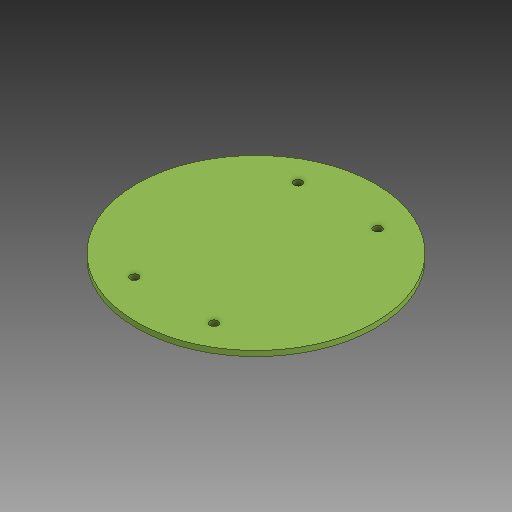
# Autodesk Inventor part: tsop_board
Saved by Autodesk Inventor 2020 (Build 240168000, 168)
## iProperties
Created: 2024-11-04
Part Number: tsop_board
Material: Медь
Document SubType Name: Modeling
Designer: Ivan
Density: 8.94 g/cm^3
Appearance: Оливково-зеленый
Mass: 133.751 g
Surface Area: 157.837 cm^2
Volume: 14.961 cm^3
Author: Ivan
Autodesk Inventor part; units mm, degrees
(part 1 of 2)
ref_plane "YZ Plane" through (0, 0, 0) normal (1, 0, 0) x (0, 1, 0)
ref_plane "XZ Plane" through (0, 0, 0) normal (0, 1, 0) x (-1, 0, 0)
ref_plane "XY Plane" through (0, 0, 0) normal (0, 0, 1) x (1, 0, 0)
sketch "Эскиз1" plane through (0, 0, 0) normal (0, 1, 0) x (-1, 0, 0)
  line L0 (44.0469, 3.6) -> (38.8469, 3.6)
  line L1 (38.8469, 3.6) -> (38.8469, -3.6)
  line L2 (38.8469, -3.6) -> (44.0469, -3.6)
  line L3 (44.0469, -3.6) -> (44.0469, 3.6)
  line L4 (0, 0) -> (38.8469, 0) construction
  circle A0 centre (0, 0) radius 41.603 construction
  line L5 (41.4469, 3.6) -> (41.4469, -3.6) construction
  line L6 (37.3982, 11.1095) -> (38.8028, 4.0478)
  line L7 (42.4983, 12.124) -> (37.3982, 11.1095)
  line L8 (43.9029, 5.0623) -> (42.4983, 12.124)
  line L9 (38.8028, 4.0478) -> (43.9029, 5.0623)
  line L10 (34.5122, 18.192) -> (37.2675, 11.5401)
  line L11 (39.3164, 20.182) -> (34.5122, 18.192)
  line L12 (42.0717, 13.5301) -> (39.3164, 20.182)
  line L13 (37.2675, 11.5401) -> (42.0717, 13.5301)
  line L14 (30.3, 24.5755) -> (34.3001, 18.5889)
  line L15 (34.6236, 27.4645) -> (30.3, 24.5755)
  line L16 (38.6237, 21.4779) -> (34.6236, 27.4645)
  line L17 (34.3001, 18.5889) -> (38.6237, 21.4779)
  line L18 (24.9233, 30.0145) -> (30.0145, 24.9233)
  line L19 (28.6003, 33.6915) -> (24.9233, 30.0145)
  line L20 (33.6915, 28.6003) -> (28.6003, 33.6915)
  line L21 (30.0145, 24.9233) -> (33.6915, 28.6003)
  line L22 (18.5889, 34.3001) -> (24.5755, 30.3)
  line L23 (21.4779, 38.6237) -> (18.5889, 34.3001)
  line L24 (27.4645, 34.6236) -> (21.4779, 38.6237)
  line L25 (24.5755, 30.3) -> (27.4645, 34.6236)
  line L26 (11.5401, 37.2675) -> (18.192, 34.5122)
  line L27 (13.5301, 42.0717) -> (11.5401, 37.2675)
  line L28 (20.182, 39.3164) -> (13.5301, 42.0717)
  line L29 (18.192, 34.5122) -> (20.182, 39.3164)
  line L30 (4.0478, 38.8028) -> (11.1095, 37.3982)
  line L31 (5.0623, 43.9029) -> (4.0478, 38.8028)
  line L32 (12.124, 42.4983) -> (5.0623, 43.9029)
  line L33 (11.1095, 37.3982) -> (12.124, 42.4983)
  line L34 (-3.6, 38.8469) -> (3.6, 38.8469)
  line L35 (-3.6, 44.0469) -> (-3.6, 38.8469)
  line L36 (3.6, 44.0469) -> (-3.6, 44.0469)
  line L37 (3.6, 38.8469) -> (3.6, 44.0469)
  line L38 (-11.1095, 37.3982) -> (-4.0478, 38.8028)
  line L39 (-12.124, 42.4983) -> (-11.1095, 37.3982)
  line L40 (-5.0623, 43.9029) -> (-12.124, 42.4983)
  line L41 (-4.0478, 38.8028) -> (-5.0623, 43.9029)
  line L42 (-18.192, 34.5122) -> (-11.5401, 37.2675)
  line L43 (-20.182, 39.3164) -> (-18.192, 34.5122)
  line L44 (-13.5301, 42.0717) -> (-20.182, 39.3164)
  line L45 (-11.5401, 37.2675) -> (-13.5301, 42.0717)
  line L46 (-24.5755, 30.3) -> (-18.5889, 34.3001)
  line L47 (-27.4645, 34.6236) -> (-24.5755, 30.3)
  line L48 (-21.4779, 38.6237) -> (-27.4645, 34.6236)
  line L49 (-18.5889, 34.3001) -> (-21.4779, 38.6237)
  line L50 (-30.0145, 24.9233) -> (-24.9233, 30.0145)
  line L51 (-33.6915, 28.6003) -> (-30.0145, 24.9233)
  line L52 (-28.6003, 33.6915) -> (-33.6915, 28.6003)
  line L53 (-24.9233, 30.0145) -> (-28.6003, 33.6915)
  line L54 (-34.3001, 18.5889) -> (-30.3, 24.5755)
  line L55 (-38.6237, 21.4779) -> (-34.3001, 18.5889)
  line L56 (-34.6236, 27.4645) -> (-38.6237, 21.4779)
  line L57 (-30.3, 24.5755) -> (-34.6236, 27.4645)
  line L58 (-37.2675, 11.5401) -> (-34.5122, 18.192)
  line L59 (-42.0717, 13.5301) -> (-37.2675, 11.5401)
  line L60 (-39.3164, 20.182) -> (-42.0717, 13.5301)
  line L61 (-34.5122, 18.192) -> (-39.3164, 20.182)
  line L62 (-38.8028, 4.0478) -> (-37.3982, 11.1095)
  line L63 (-43.9029, 5.0623) -> (-38.8028, 4.0478)
  line L64 (-42.4983, 12.124) -> (-43.9029, 5.0623)
  line L65 (-37.3982, 11.1095) -> (-42.4983, 12.124)
  line L66 (-38.8469, -3.6) -> (-38.8469, 3.6)
  line L67 (-44.0469, -3.6) -> (-38.8469, -3.6)
  line L68 (-44.0469, 3.6) -> (-44.0469, -3.6)
  line L69 (-38.8469, 3.6) -> (-44.0469, 3.6)
  line L70 (-37.3982, -11.1095) -> (-38.8028, -4.0478)
  line L71 (-42.4983, -12.124) -> (-37.3982, -11.1095)
  line L72 (-43.9029, -5.0623) -> (-42.4983, -12.124)
  line L73 (-38.8028, -4.0478) -> (-43.9029, -5.0623)
  line L74 (-34.5122, -18.192) -> (-37.2675, -11.5401)
  line L75 (-39.3164, -20.182) -> (-34.5122, -18.192)
  line L76 (-42.0717, -13.5301) -> (-39.3164, -20.182)
  line L77 (-37.2675, -11.5401) -> (-42.0717, -13.5301)
  line L78 (-30.3, -24.5755) -> (-34.3001, -18.5889)
  line L79 (-34.6236, -27.4645) -> (-30.3, -24.5755)
  line L80 (-38.6237, -21.4779) -> (-34.6236, -27.4645)
  line L81 (-34.3001, -18.5889) -> (-38.6237, -21.4779)
  line L82 (-24.9233, -30.0145) -> (-30.0145, -24.9233)
  line L83 (-28.6003, -33.6915) -> (-24.9233, -30.0145)
  line L84 (-33.6915, -28.6003) -> (-28.6003, -33.6915)
  line L85 (-30.0145, -24.9233) -> (-33.6915, -28.6003)
  line L86 (-18.5889, -34.3001) -> (-24.5755, -30.3)
  line L87 (-21.4779, -38.6237) -> (-18.5889, -34.3001)
  line L88 (-27.4645, -34.6236) -> (-21.4779, -38.6237)
  line L89 (-24.5755, -30.3) -> (-27.4645, -34.6236)
  line L90 (-11.5401, -37.2675) -> (-18.192, -34.5122)
  line L91 (-13.5301, -42.0717) -> (-11.5401, -37.2675)
  line L92 (-20.182, -39.3164) -> (-13.5301, -42.0717)
  line L93 (-18.192, -34.5122) -> (-20.182, -39.3164)
  line L94 (-4.0478, -38.8028) -> (-11.1095, -37.3982)
  line L95 (-5.0623, -43.9029) -> (-4.0478, -38.8028)
  line L96 (-12.124, -42.4983) -> (-5.0623, -43.9029)
  line L97 (-11.1095, -37.3982) -> (-12.124, -42.4983)
  line L98 (3.6, -38.8469) -> (-3.6, -38.8469)
  line L99 (3.6, -44.0469) -> (3.6, -38.8469)
  line L100 (-3.6, -44.0469) -> (3.6, -44.0469)
  line L101 (-3.6, -38.8469) -> (-3.6, -44.0469)
  line L102 (11.1095, -37.3982) -> (4.0478, -38.8028)
  line L103 (12.124, -42.4983) -> (11.1095, -37.3982)
  line L104 (5.0623, -43.9029) -> (12.124, -42.4983)
  line L105 (4.0478, -38.8028) -> (5.0623, -43.9029)
  line L106 (18.192, -34.5122) -> (11.5401, -37.2675)
  line L107 (20.182, -39.3164) -> (18.192, -34.5122)
  line L108 (13.5301, -42.0717) -> (20.182, -39.3164)
  line L109 (11.5401, -37.2675) -> (13.5301, -42.0717)
  line L110 (24.5755, -30.3) -> (18.5889, -34.3001)
  line L111 (27.4645, -34.6236) -> (24.5755, -30.3)
  line L112 (21.4779, -38.6237) -> (27.4645, -34.6236)
  line L113 (18.5889, -34.3001) -> (21.4779, -38.6237)
  line L114 (30.0145, -24.9233) -> (24.9233, -30.0145)
  line L115 (33.6915, -28.6003) -> (30.0145, -24.9233)
  line L116 (28.6003, -33.6915) -> (33.6915, -28.6003)
  line L117 (24.9233, -30.0145) -> (28.6003, -33.6915)
  line L118 (34.3001, -18.5889) -> (30.3, -24.5755)
  line L119 (38.6237, -21.4779) -> (34.3001, -18.5889)
  line L120 (34.6236, -27.4645) -> (38.6237, -21.4779)
  line L121 (30.3, -24.5755) -> (34.6236, -27.4645)
  line L122 (37.2675, -11.5401) -> (34.5122, -18.192)
  line L123 (42.0717, -13.5301) -> (37.2675, -11.5401)
  line L124 (39.3164, -20.182) -> (42.0717, -13.5301)
  line L125 (34.5122, -18.192) -> (39.3164, -20.182)
  line L126 (38.8028, -4.0478) -> (37.3982, -11.1095)
  line L127 (43.9029, -5.0623) -> (38.8028, -4.0478)
  line L128 (42.4983, -12.124) -> (43.9029, -5.0623)
  line L129 (37.3982, -11.1095) -> (42.4983, -12.124)
  line L130 (38.8028, 4.0478) -> (38.8469, 3.6) construction
  line L131 (38.8469, 3.6) -> (43.9777, 4.1053) construction
  line L132 (43.9029, 5.0623) -> (37.3982, 11.1095) construction
  line L133 (42.4983, 12.124) -> (38.8028, 4.0478) construction
  circle A1 centre (0, 0) radius 41.4469 construction
  line L134 (39.3164, 20.182) -> (37.2675, 11.5401) construction
  line L135 (34.5122, 18.192) -> (42.0717, 13.5301) construction
  line L136 (38.292, 15.8611) -> (0, 0) construction
  line L137 (0, 0) -> (40.6505, 8.0859) construction
  point P0 (41.603, 0)
  point P1 (38.1005, 7.5787)
  point P2 (39.9482, 11.6167)
  point P3 (41.3529, 4.5551)
  point P4 (35.8899, 14.8661)
  point P5 (36.9143, 19.187)
  point P6 (39.6696, 12.5351)
  point P7 (32.3, 21.5822)
  point P8 (32.4618, 26.02)
  point P9 (36.4619, 20.0334)
  point P10 (27.4689, 27.4689)
  point P11 (26.7618, 31.853)
  point P12 (31.853, 26.7618)
  point P13 (21.5822, 32.3)
  point P14 (20.0334, 36.4619)
  point P15 (26.02, 32.4618)
  point P16 (14.8661, 35.8899)
  point P17 (12.5351, 39.6696)
  point P18 (19.187, 36.9143)
  point P19 (7.5787, 38.1005)
  point P20 (4.5551, 41.3529)
  point P21 (11.6167, 39.9482)
  point P22 (0, 38.8469)
  point P23 (-3.6, 41.4469)
  point P24 (3.6, 41.4469)
  point P25 (-7.5787, 38.1005)
  point P26 (-11.6167, 39.9482)
  point P27 (-4.5551, 41.3529)
  point P28 (-14.8661, 35.8899)
  point P29 (-19.187, 36.9143)
  point P30 (-12.5351, 39.6696)
  point P31 (-21.5822, 32.3)
  point P32 (-26.02, 32.4618)
  point P33 (-20.0334, 36.4619)
  point P34 (-27.4689, 27.4689)
  point P35 (-31.853, 26.7618)
  point P36 (-26.7618, 31.853)
  point P37 (-32.3, 21.5822)
  point P38 (-36.4619, 20.0334)
  point P39 (-32.4618, 26.02)
  point P40 (-35.8899, 14.8661)
  point P41 (-39.6696, 12.5351)
  point P42 (-36.9143, 19.187)
  point P43 (-38.1005, 7.5787)
  point P44 (-41.3529, 4.5551)
  point P45 (-39.9482, 11.6167)
  point P46 (-38.8469, 0)
  point P47 (-41.4469, -3.6)
  point P48 (-41.4469, 3.6)
  point P49 (-38.1005, -7.5787)
  point P50 (-39.9482, -11.6167)
  point P51 (-41.3529, -4.5551)
  point P52 (-35.8899, -14.8661)
  point P53 (-36.9143, -19.187)
  point P54 (-39.6696, -12.5351)
  point P55 (-32.3, -21.5822)
  point P56 (-32.4618, -26.02)
  point P57 (-36.4619, -20.0334)
  point P58 (-27.4689, -27.4689)
  point P59 (-26.7618, -31.853)
  point P60 (-31.853, -26.7618)
  point P61 (-21.5822, -32.3)
  point P62 (-20.0334, -36.4619)
  point P63 (-26.02, -32.4618)
  point P64 (-14.8661, -35.8899)
  point P65 (-12.5351, -39.6696)
  point P66 (-19.187, -36.9143)
  point P67 (-7.5787, -38.1005)
  point P68 (-4.5551, -41.3529)
  point P69 (-11.6167, -39.9482)
  point P70 (0, -38.8469)
  point P71 (3.6, -41.4469)
  point P72 (-3.6, -41.4469)
  point P73 (7.5787, -38.1005)
  point P74 (11.6167, -39.9482)
  point P75 (4.5551, -41.3529)
  point P76 (14.8661, -35.8899)
  point P77 (19.187, -36.9143)
  point P78 (12.5351, -39.6696)
  point P79 (21.5822, -32.3)
  point P80 (26.02, -32.4618)
  point P81 (20.0334, -36.4619)
  point P82 (27.4689, -27.4689)
  point P83 (31.853, -26.7618)
  point P84 (26.7618, -31.853)
  point P85 (32.3, -21.5822)
  point P86 (36.4619, -20.0334)
  point P87 (32.4618, -26.02)
  point P88 (35.8899, -14.8661)
  point P89 (39.6696, -12.5351)
  point P90 (36.9143, -19.187)
  point P91 (38.1005, -7.5787)
  point P92 (41.3529, -4.5551)
  point P93 (39.9482, -11.6167)
sketch "Эскиз3" plane through (0, 0, 0) normal (0, 1, 0) x (-1, 0, 0)
  line L0 (38.8028, 4.0478) -> (38.8469, 3.6) construction
  line L1 (38.8249, 3.8239) -> (46.4311, 4.5731) construction
  line L2 (44.0469, -3.6) -> (44.0469, 3.6)
  line L3 (44.0469, -0.05) -> (44.0469, 0.05)
  line L4 (44.0469, 2.45) -> (45.2469, 2.45) construction
  arc A0 (44.0469, 0.05) -> (45.2469, 2.45) centre (42.2469, 2.45) ccw
  line L5 (45.2469, 2.45) -> (45.2469, 0) construction
  line L6 (0, 0) -> (38.8469, 0) construction
  arc A1 (45.2469, -2.45) -> (44.0469, -0.05) centre (42.2469, -2.45) ccw
  arc A2 (43.1908, 8.6422) -> (43.8996, 11.2302) centre (40.9572, 10.6449) ccw
  arc A3 (44.8555, 6.4243) -> (43.2103, 8.5441) centre (41.9131, 5.839) ccw
  line L7 (43.2103, 8.5441) -> (43.1908, 8.6422)
  arc A4 (40.6749, 16.9022) -> (40.8651, 19.5788) centre (38.0935, 18.4307) ccw
  arc A5 (42.7403, 15.0517) -> (40.7132, 16.8098) centre (39.9686, 13.9037) ccw
  line L8 (40.7132, 16.8098) -> (40.6749, 16.9022)
  arc A6 (36.5959, 24.5127) -> (36.2603, 27.1749) centre (33.7659, 25.5082) ccw
  arc A7 (38.9826, 23.1007) -> (36.6515, 24.4296) centre (36.4882, 21.434) ccw
  line L9 (36.6515, 24.4296) -> (36.5959, 24.5127)
  arc A8 (31.1105, 31.1812) -> (30.262, 33.7268) centre (28.1407, 31.6055) ccw
  arc A9 (33.7268, 30.262) -> (31.1812, 31.1105) centre (31.6055, 28.1407) ccw
  line L10 (31.1812, 31.1105) -> (31.1105, 31.1812)
  arc A10 (24.4296, 36.6515) -> (23.1007, 38.9826) centre (21.434, 36.4882) ccw
  arc A11 (27.1749, 36.2603) -> (24.5127, 36.5959) centre (25.5082, 33.7659) ccw
  line L11 (24.5127, 36.5959) -> (24.4296, 36.6515)
  arc A12 (16.8098, 40.7132) -> (15.0517, 42.7403) centre (13.9037, 39.9686) ccw
  arc A13 (19.5788, 40.8651) -> (16.9022, 40.6749) centre (18.4307, 38.0935) ccw
  line L12 (16.9022, 40.6749) -> (16.8098, 40.7132)
  arc A14 (8.5441, 43.2103) -> (6.4243, 44.8555) centre (5.839, 41.9131) ccw
  arc A15 (11.2302, 43.8996) -> (8.6422, 43.1908) centre (10.6449, 40.9572) ccw
  line L13 (8.6422, 43.1908) -> (8.5441, 43.2103)
  arc A16 (-0.05, 44.0469) -> (-2.45, 45.2469) centre (-2.45, 42.2469) ccw
  arc A17 (2.45, 45.2469) -> (0.05, 44.0469) centre (2.45, 42.2469) ccw
  line L14 (0.05, 44.0469) -> (-0.05, 44.0469)
  arc A18 (-8.6422, 43.1908) -> (-11.2302, 43.8996) centre (-10.6449, 40.9572) ccw
  arc A19 (-6.4243, 44.8555) -> (-8.5441, 43.2103) centre (-5.839, 41.9131) ccw
  line L15 (-8.5441, 43.2103) -> (-8.6422, 43.1908)
  arc A20 (-16.9022, 40.6749) -> (-19.5788, 40.8651) centre (-18.4307, 38.0935) ccw
  arc A21 (-15.0517, 42.7403) -> (-16.8098, 40.7132) centre (-13.9037, 39.9686) ccw
  line L16 (-16.8098, 40.7132) -> (-16.9022, 40.6749)
  arc A22 (-24.5127, 36.5959) -> (-27.1749, 36.2603) centre (-25.5082, 33.7659) ccw
  arc A23 (-23.1007, 38.9826) -> (-24.4296, 36.6515) centre (-21.434, 36.4882) ccw
  line L17 (-24.4296, 36.6515) -> (-24.5127, 36.5959)
  arc A24 (-31.1812, 31.1105) -> (-33.7268, 30.262) centre (-31.6055, 28.1407) ccw
  arc A25 (-30.262, 33.7268) -> (-31.1105, 31.1812) centre (-28.1407, 31.6055) ccw
  line L18 (-31.1105, 31.1812) -> (-31.1812, 31.1105)
  arc A26 (-36.6515, 24.4296) -> (-38.9826, 23.1007) centre (-36.4882, 21.434) ccw
  arc A27 (-36.2603, 27.1749) -> (-36.5959, 24.5127) centre (-33.7659, 25.5082) ccw
  line L19 (-36.5959, 24.5127) -> (-36.6515, 24.4296)
  arc A28 (-40.7132, 16.8098) -> (-42.7403, 15.0517) centre (-39.9686, 13.9037) ccw
  arc A29 (-40.8651, 19.5788) -> (-40.6749, 16.9022) centre (-38.0935, 18.4307) ccw
  line L20 (-40.6749, 16.9022) -> (-40.7132, 16.8098)
  arc A30 (-43.2103, 8.5441) -> (-44.8555, 6.4243) centre (-41.9131, 5.839) ccw
  arc A31 (-43.8996, 11.2302) -> (-43.1908, 8.6422) centre (-40.9572, 10.6449) ccw
  line L21 (-43.1908, 8.6422) -> (-43.2103, 8.5441)
  arc A32 (-44.0469, -0.05) -> (-45.2469, -2.45) centre (-42.2469, -2.45) ccw
  arc A33 (-45.2469, 2.45) -> (-44.0469, 0.05) centre (-42.2469, 2.45) ccw
  line L22 (-44.0469, 0.05) -> (-44.0469, -0.05)
  arc A34 (-43.1908, -8.6422) -> (-43.8996, -11.2302) centre (-40.9572, -10.6449) ccw
  arc A35 (-44.8555, -6.4243) -> (-43.2103, -8.5441) centre (-41.9131, -5.839) ccw
  line L23 (-43.2103, -8.5441) -> (-43.1908, -8.6422)
  arc A36 (-40.6749, -16.9022) -> (-40.8651, -19.5788) centre (-38.0935, -18.4307) ccw
  arc A37 (-42.7403, -15.0517) -> (-40.7132, -16.8098) centre (-39.9686, -13.9037) ccw
  line L24 (-40.7132, -16.8098) -> (-40.6749, -16.9022)
  arc A38 (-36.5959, -24.5127) -> (-36.2603, -27.1749) centre (-33.7659, -25.5082) ccw
  arc A39 (-38.9826, -23.1007) -> (-36.6515, -24.4296) centre (-36.4882, -21.434) ccw
  line L25 (-36.6515, -24.4296) -> (-36.5959, -24.5127)
  arc A40 (-31.1105, -31.1812) -> (-30.262, -33.7268) centre (-28.1407, -31.6055) ccw
  arc A41 (-33.7268, -30.262) -> (-31.1812, -31.1105) centre (-31.6055, -28.1407) ccw
  line L26 (-31.1812, -31.1105) -> (-31.1105, -31.1812)
  arc A42 (-24.4296, -36.6515) -> (-23.1007, -38.9826) centre (-21.434, -36.4882) ccw
  arc A43 (-27.1749, -36.2603) -> (-24.5127, -36.5959) centre (-25.5082, -33.7659) ccw
  line L27 (-24.5127, -36.5959) -> (-24.4296, -36.6515)
  arc A44 (-16.8098, -40.7132) -> (-15.0517, -42.7403) centre (-13.9037, -39.9686) ccw
  arc A45 (-19.5788, -40.8651) -> (-16.9022, -40.6749) centre (-18.4307, -38.0935) ccw
  line L28 (-16.9022, -40.6749) -> (-16.8098, -40.7132)
  arc A46 (-8.5441, -43.2103) -> (-6.4243, -44.8555) centre (-5.839, -41.9131) ccw
  arc A47 (-11.2302, -43.8996) -> (-8.6422, -43.1908) centre (-10.6449, -40.9572) ccw
  line L29 (-8.6422, -43.1908) -> (-8.5441, -43.2103)
  arc A48 (0.05, -44.0469) -> (2.45, -45.2469) centre (2.45, -42.2469) ccw
  arc A49 (-2.45, -45.2469) -> (-0.05, -44.0469) centre (-2.45, -42.2469) ccw
  line L30 (-0.05, -44.0469) -> (0.05, -44.0469)
  arc A50 (8.6422, -43.1908) -> (11.2302, -43.8996) centre (10.6449, -40.9572) ccw
  arc A51 (6.4243, -44.8555) -> (8.5441, -43.2103) centre (5.839, -41.9131) ccw
  line L31 (8.5441, -43.2103) -> (8.6422, -43.1908)
  arc A52 (16.9022, -40.6749) -> (19.5788, -40.8651) centre (18.4307, -38.0935) ccw
  arc A53 (15.0517, -42.7403) -> (16.8098, -40.7132) centre (13.9037, -39.9686) ccw
  line L32 (16.8098, -40.7132) -> (16.9022, -40.6749)
  arc A54 (24.5127, -36.5959) -> (27.1749, -36.2603) centre (25.5082, -33.7659) ccw
  arc A55 (23.1007, -38.9826) -> (24.4296, -36.6515) centre (21.434, -36.4882) ccw
  line L33 (24.4296, -36.6515) -> (24.5127, -36.5959)
  arc A56 (31.1812, -31.1105) -> (33.7268, -30.262) centre (31.6055, -28.1407) ccw
  arc A57 (30.262, -33.7268) -> (31.1105, -31.1812) centre (28.1407, -31.6055) ccw
  line L34 (31.1105, -31.1812) -> (31.1812, -31.1105)
  arc A58 (36.6515, -24.4296) -> (38.9826, -23.1007) centre (36.4882, -21.434) ccw
  arc A59 (36.2603, -27.1749) -> (36.5959, -24.5127) centre (33.7659, -25.5082) ccw
  line L35 (36.5959, -24.5127) -> (36.6515, -24.4296)
  arc A60 (40.7132, -16.8098) -> (42.7403, -15.0517) centre (39.9686, -13.9037) ccw
  arc A61 (40.8651, -19.5788) -> (40.6749, -16.9022) centre (38.0935, -18.4307) ccw
  line L36 (40.6749, -16.9022) -> (40.7132, -16.8098)
  arc A62 (43.2103, -8.5441) -> (44.8555, -6.4243) centre (41.9131, -5.839) ccw
  arc A63 (43.8996, -11.2302) -> (43.1908, -8.6422) centre (40.9572, -10.6449) ccw
  line L37 (43.1908, -8.6422) -> (43.2103, -8.5441)
  arc A64 (45.2469, 2.45) -> (44.8555, 6.4243) centre (0, 0) ccw
  arc A65 (43.8996, 11.2302) -> (42.7403, 15.0517) centre (0, 0) ccw
  arc A66 (40.8651, 19.5788) -> (38.9826, 23.1007) centre (0, 0) ccw
  arc A67 (36.2603, 27.1749) -> (33.7268, 30.262) centre (0, 0) ccw
  arc A68 (30.262, 33.7268) -> (27.1749, 36.2603) centre (0, 0) ccw
  arc A69 (23.1007, 38.9826) -> (19.5788, 40.8651) centre (0, 0) ccw
  arc A70 (15.0517, 42.7403) -> (11.2302, 43.8996) centre (0, 0) ccw
  arc A71 (6.4243, 44.8555) -> (2.45, 45.2469) centre (0, 0) ccw
  arc A72 (-2.45, 45.2469) -> (-6.4243, 44.8555) centre (0, 0) ccw
  arc A73 (-11.2302, 43.8996) -> (-15.0517, 42.7403) centre (0, 0) ccw
  arc A74 (-19.5788, 40.8651) -> (-23.1007, 38.9826) centre (0, 0) ccw
  arc A75 (-27.1749, 36.2603) -> (-30.262, 33.7268) centre (0, 0) ccw
  arc A76 (-33.7268, 30.262) -> (-36.2603, 27.1749) centre (0, 0) ccw
  arc A77 (-38.9826, 23.1007) -> (-40.8651, 19.5788) centre (0, 0) ccw
  arc A78 (-42.7403, 15.0517) -> (-43.8996, 11.2302) centre (0, 0) ccw
  arc A79 (-44.8555, 6.4243) -> (-45.2469, 2.45) centre (0, 0) ccw
  arc A80 (-45.2469, -2.45) -> (-44.8555, -6.4243) centre (0, 0) ccw
  arc A81 (-43.8996, -11.2302) -> (-42.7403, -15.0517) centre (0, 0) ccw
  arc A82 (-40.8651, -19.5788) -> (-38.9826, -23.1007) centre (0, 0) ccw
  arc A83 (-36.2603, -27.1749) -> (-33.7268, -30.262) centre (0, 0) ccw
  arc A84 (-30.262, -33.7268) -> (-27.1749, -36.2603) centre (0, 0) ccw
  arc A85 (-23.1007, -38.9826) -> (-19.5788, -40.8651) centre (0, 0) ccw
  arc A86 (-15.0517, -42.7403) -> (-11.2302, -43.8996) centre (0, 0) ccw
  arc A87 (-6.4243, -44.8555) -> (-2.45, -45.2469) centre (0, 0) ccw
  arc A88 (2.45, -45.2469) -> (6.4243, -44.8555) centre (0, 0) ccw
  arc A89 (11.2302, -43.8996) -> (15.0517, -42.7403) centre (0, 0) ccw
  arc A90 (19.5788, -40.8651) -> (23.1007, -38.9826) centre (0, 0) ccw
  arc A91 (27.1749, -36.2603) -> (30.262, -33.7268) centre (0, 0) ccw
  arc A92 (33.7268, -30.262) -> (36.2603, -27.1749) centre (0, 0) ccw
  arc A93 (38.9826, -23.1007) -> (40.8651, -19.5788) centre (0, 0) ccw
  arc A94 (42.7403, -15.0517) -> (43.8996, -11.2302) centre (0, 0) ccw
  arc A95 (44.8555, -6.4243) -> (45.2469, -2.45) centre (0, 0) ccw
  circle A96 centre (0, 0) radius 36.8469
  line L38 (38.8469, 3.6) -> (38.8469, -3.6)
  point P0 (44.0469, 0)
  point P1 (43.2006, 8.5931)
  point P2 (40.6941, 16.856)
  point P3 (36.6237, 24.4712)
  point P4 (31.1459, 31.1459)
  point P5 (24.4712, 36.6237)
  point P6 (16.856, 40.6941)
  point P7 (8.5931, 43.2006)
  point P8 (0, 44.0469)
  point P9 (-8.5931, 43.2006)
  point P10 (-16.856, 40.6941)
  point P11 (-24.4712, 36.6237)
  point P12 (-31.1459, 31.1459)
  point P13 (-36.6237, 24.4712)
  point P14 (-40.6941, 16.856)
  point P15 (-43.2006, 8.5931)
  point P16 (-44.0469, 0)
  point P17 (-43.2006, -8.5931)
  point P18 (-40.6941, -16.856)
  point P19 (-36.6237, -24.4712)
  point P20 (-31.1459, -31.1459)
  point P21 (-24.4712, -36.6237)
  point P22 (-16.856, -40.6941)
  point P23 (-8.5931, -43.2006)
  point P24 (0, -44.0469)
  point P25 (8.5931, -43.2006)
  point P26 (16.856, -40.6941)
  point P27 (24.4712, -36.6237)
  point P28 (31.1459, -31.1459)
  point P29 (36.6237, -24.4712)
  point P30 (40.6941, -16.856)
  point P31 (43.2006, -8.5931)
  point P32 (36.8469, 0)
  point P33 (44.8555, -6.4243)
  point P34 (45.2469, -2.45)
  point P35 (44.0469, -0.05)
  point P36 (44.0469, 0.05)
  point P37 (43.8996, 11.2302)
  point P38 (42.7403, 15.0517)
  point P39 (40.8651, 19.5788)
  point P40 (38.9826, 23.1007)
  point P41 (36.2603, 27.1749)
  point P42 (33.7268, 30.262)
  point P43 (30.262, 33.7268)
  point P44 (27.1749, 36.2603)
  point P45 (23.1007, 38.9826)
  point P46 (19.5788, 40.8651)
  point P47 (15.0517, 42.7403)
  point P48 (11.2302, 43.8996)
  point P49 (6.4243, 44.8555)
  point P50 (2.45, 45.2469)
  point P51 (-2.45, 45.2469)
  point P52 (-6.4243, 44.8555)
  point P53 (-11.2302, 43.8996)
  point P54 (-15.0517, 42.7403)
  point P55 (-19.5788, 40.8651)
  point P56 (-23.1007, 38.9826)
  point P57 (-27.1749, 36.2603)
  point P58 (-30.262, 33.7268)
  point P59 (-33.7268, 30.262)
  point P60 (-36.2603, 27.1749)
  point P61 (-38.9826, 23.1007)
  point P62 (-40.8651, 19.5788)
  point P63 (-42.7403, 15.0517)
  point P64 (-43.8996, 11.2302)
  point P65 (-44.8555, 6.4243)
  point P66 (-45.2469, 2.45)
  point P67 (-45.2469, -2.45)
  point P68 (-44.8555, -6.4243)
  point P69 (-43.8996, -11.2302)
  point P70 (-42.7403, -15.0517)
  point P71 (-40.8651, -19.5788)
  point P72 (-38.9826, -23.1007)
  point P73 (-36.2603, -27.1749)
  point P74 (-33.7268, -30.262)
  point P75 (-30.262, -33.7268)
  point P76 (-27.1749, -36.2603)
  point P77 (-23.1007, -38.9826)
  point P78 (-19.5788, -40.8651)
  point P79 (-15.0517, -42.7403)
  point P80 (-11.2302, -43.8996)
  point P81 (-6.4243, -44.8555)
  point P82 (-2.45, -45.2469)
  point P83 (2.45, -45.2469)
  point P84 (6.4243, -44.8555)
  point P85 (11.2302, -43.8996)
  point P86 (15.0517, -42.7403)
  point P87 (19.5788, -40.8651)
  point P88 (23.1007, -38.9826)
  point P89 (27.1749, -36.2603)
  point P90 (30.262, -33.7268)
  point P91 (33.7268, -30.262)
  point P92 (36.2603, -27.1749)
  point P93 (38.9826, -23.1007)
  point P94 (40.8651, -19.5788)
  point P95 (42.7403, -15.0517)
  point P96 (43.8996, -11.2302)
sketch "Эскиз7" plane through (0, 0.5, 0) normal (0, 1, 0) x (1, 0, 0)
  circle A0 centre (0, 0) radius 36.8469
  circle A1 centre (15.1, -31) radius 1.65
  circle A2 centre (0, -22.6275) radius 2
  circle A3 centre (-15.1, -31) radius 1.65
  circle A4 centre (-15.1, 31) radius 1.65
  circle A5 centre (0, 22.6275) radius 2
  circle A6 centre (15.1, 31) radius 1.65
  circle A7 centre (-15.1, -31) radius 3.25 construction
  circle A8 centre (15.1, -31) radius 1.65
  circle A9 centre (15.1, -31) radius 3.25 construction
  circle A10 centre (15.1, 31) radius 3.05 construction
  circle A11 centre (15.1, 31) radius 3.25 construction
  circle A12 centre (-15.1, 31) radius 1.65
  circle A13 centre (-15.1, 31) radius 3.25 construction
  circle A14 centre (0, 0) radius 36.8469
  line L0 (-13.9766, -34.0933) -> (0, -26.3437)
  line L1 (-20.7761, -30.4311) -> (-1.576, -19.7852)
  line L2 (13.9766, -34.0933) -> (-1.576, -25.4698)
  line L3 (20.7761, -30.4311) -> (1.576, -19.7852)
  line L4 (-15.1, -31) -> (-9.8654, -28.0975) construction
  line L5 (15.1, -31) -> (8.9364, -27.5825) construction
  circle A15 centre (0, -22.6275) radius 3.25
  line L6 (0, 0) -> (-36.8469, 0) construction
  line L7 (-20.7761, 30.4311) -> (-1.576, 19.7852)
  line L8 (-13.9766, 34.0933) -> (0, 26.3437)
  line L9 (13.9766, 34.0933) -> (-1.576, 25.4698)
  line L10 (20.7761, 30.4311) -> (1.576, 19.7852)
  circle A16 centre (0, 22.6275) radius 3.25
  circle A17 centre (-15.1, -31) radius 1.65
  circle A18 centre (-15.1, -31) radius 3.05
  circle A19 centre (15.1, -31) radius 3.05
  circle A20 centre (15.1, 31) radius 3.05
  circle A21 centre (-15.1, 31) radius 3.05
  circle A22 centre (-15.1, -31) radius 3.05
  point P0 (20.7761, 30.4311)
  point P1 (-13.9766, 34.0933)
  point P2 (-20.7761, 30.4311)
  point P3 (-20.7761, -30.4311)
  point P4 (-13.9766, -34.0933)
  point P5 (13.9766, -34.0933)
  point P6 (20.7761, -30.4311)
sketch "Эскиз32" plane through (0, -2, 0) normal (0, -1, 0) x (1, 0, 0)
  line L0 (-6.8284, -25.6275) -> (-22.888, -25.6275)
  arc A0 (-23.5951, -25.3346) -> (-22.888, -25.6275) centre (-22.888, -24.6275) ccw
  line L1 (-23.5951, -25.3346) -> (-28.0726, -20.8571)
  arc A1 (-27.3655, -19.15) -> (-28.0726, -20.8571) centre (-27.3655, -20.15) ccw
  line L2 (-27.3655, -19.15) -> (-11.3059, -19.15)
  arc A2 (-10.5988, -19.4429) -> (-11.3059, -19.15) centre (-11.3059, -20.15) ccw
  line L3 (-10.5988, -19.4429) -> (-6.1213, -23.9204)
  arc A3 (-6.8284, -25.6275) -> (-6.1213, -23.9204) centre (-6.8284, -24.6275) ccw
  line L4 (11.3059, -19.15) -> (27.3655, -19.15)
  arc A4 (28.0726, -20.8571) -> (27.3655, -19.15) centre (27.3655, -20.15) ccw
  line L5 (28.0726, -20.8571) -> (23.5951, -25.3346)
  arc A5 (22.888, -25.6275) -> (23.5951, -25.3346) centre (22.888, -24.6275) ccw
  line L6 (22.888, -25.6275) -> (6.8284, -25.6275)
  arc A6 (6.1213, -23.9204) -> (6.8284, -25.6275) centre (6.8284, -24.6275) ccw
  line L7 (6.1213, -23.9204) -> (10.5988, -19.4429)
  arc A7 (11.3059, -19.15) -> (10.5988, -19.4429) centre (11.3059, -20.15) ccw
  line L8 (-22.888, 25.6275) -> (-6.8284, 25.6275)
  arc A8 (-6.1213, 23.9204) -> (-6.8284, 25.6275) centre (-6.8284, 24.6275) ccw
  line L9 (-6.1213, 23.9204) -> (-10.5988, 19.4429)
  arc A9 (-11.3059, 19.15) -> (-10.5988, 19.4429) centre (-11.3059, 20.15) ccw
  line L10 (-11.3059, 19.15) -> (-27.3655, 19.15)
  arc A10 (-28.0726, 20.8571) -> (-27.3655, 19.15) centre (-27.3655, 20.15) ccw
  line L11 (-28.0726, 20.8571) -> (-23.5951, 25.3346)
  arc A11 (-22.888, 25.6275) -> (-23.5951, 25.3346) centre (-22.888, 24.6275) ccw
  line L12 (27.3655, 19.15) -> (11.3059, 19.15)
  arc A12 (10.5988, 19.4429) -> (11.3059, 19.15) centre (11.3059, 20.15) ccw
  line L13 (10.5988, 19.4429) -> (6.1213, 23.9204)
  arc A13 (6.8284, 25.6275) -> (6.1213, 23.9204) centre (6.8284, 24.6275) ccw
  line L14 (6.8284, 25.6275) -> (22.888, 25.6275)
  arc A14 (23.5951, 25.3346) -> (22.888, 25.6275) centre (22.888, 24.6275) ccw
  line L15 (23.5951, 25.3346) -> (28.0726, 20.8571)
  arc A15 (27.3655, 19.15) -> (28.0726, 20.8571) centre (27.3655, 20.15) ccw
  circle A16 centre (-15.1, -31) radius 3.05
  circle A17 centre (-15.1, 31) radius 3.05
  circle A18 centre (0, -22.6275) radius 2
  circle A19 centre (0, 22.6275) radius 2
  line L16 (-44.0469, 0.05) -> (-44.0469, -0.05)
  arc A20 (-44.0469, -0.05) -> (-45.2469, -2.45) centre (-42.2469, -2.45) ccw
  arc A21 (-45.2469, -2.45) -> (-44.8555, -6.4243) centre (0, 0) ccw
  arc A22 (-44.8555, -6.4243) -> (-43.2103, -8.5441) centre (-41.9131, -5.839) ccw
  line L17 (-43.2103, -8.5441) -> (-43.1908, -8.6422)
  arc A23 (-43.1908, -8.6422) -> (-43.8996, -11.2302) centre (-40.9572, -10.6449) ccw
  arc A24 (-43.8996, -11.2302) -> (-42.7403, -15.0517) centre (0, 0) ccw
  arc A25 (-42.7403, -15.0517) -> (-40.7132, -16.8098) centre (-39.9686, -13.9037) ccw
  line L18 (-40.7132, -16.8098) -> (-40.6749, -16.9022)
  arc A26 (-40.6749, -16.9022) -> (-40.8651, -19.5788) centre (-38.0935, -18.4307) ccw
  arc A27 (-40.8651, -19.5788) -> (-38.9826, -23.1007) centre (0, 0) ccw
  arc A28 (-38.9826, -23.1007) -> (-36.6515, -24.4296) centre (-36.4882, -21.434) ccw
  line L19 (-36.6515, -24.4296) -> (-36.5959, -24.5127)
  arc A29 (-36.5959, -24.5127) -> (-36.2603, -27.1749) centre (-33.7659, -25.5082) ccw
  arc A30 (-36.2603, -27.1749) -> (-33.7268, -30.262) centre (0, 0) ccw
  arc A31 (-33.7268, -30.262) -> (-31.1812, -31.1105) centre (-31.6055, -28.1407) ccw
  line L20 (-31.1812, -31.1105) -> (-31.1105, -31.1812)
  arc A32 (-31.1105, -31.1812) -> (-30.262, -33.7268) centre (-28.1407, -31.6055) ccw
  arc A33 (-30.262, -33.7268) -> (-27.1749, -36.2603) centre (0, 0) ccw
  arc A34 (-27.1749, -36.2603) -> (-24.5127, -36.5959) centre (-25.5082, -33.7659) ccw
  line L21 (-24.5127, -36.5959) -> (-24.4296, -36.6515)
  arc A35 (-24.4296, -36.6515) -> (-23.1007, -38.9826) centre (-21.434, -36.4882) ccw
  arc A36 (-23.1007, -38.9826) -> (-19.5788, -40.8651) centre (0, 0) ccw
  arc A37 (-19.5788, -40.8651) -> (-16.9022, -40.6749) centre (-18.4307, -38.0935) ccw
  line L22 (-16.9022, -40.6749) -> (-16.8098, -40.7132)
  arc A38 (-16.8098, -40.7132) -> (-15.0517, -42.7403) centre (-13.9037, -39.9686) ccw
  arc A39 (-15.0517, -42.7403) -> (-11.2302, -43.8996) centre (0, 0) ccw
  arc A40 (-11.2302, -43.8996) -> (-8.6422, -43.1908) centre (-10.6449, -40.9572) ccw
  line L23 (-8.6422, -43.1908) -> (-8.5441, -43.2103)
  arc A41 (-8.5441, -43.2103) -> (-6.4243, -44.8555) centre (-5.839, -41.9131) ccw
  arc A42 (-6.4243, -44.8555) -> (-2.45, -45.2469) centre (0, 0) ccw
  arc A43 (-2.45, -45.2469) -> (-0.05, -44.0469) centre (-2.45, -42.2469) ccw
  line L24 (-0.05, -44.0469) -> (0.05, -44.0469)
  arc A44 (0.05, -44.0469) -> (2.45, -45.2469) centre (2.45, -42.2469) ccw
  arc A45 (2.45, -45.2469) -> (6.4243, -44.8555) centre (0, 0) ccw
  arc A46 (6.4243, -44.8555) -> (8.5441, -43.2103) centre (5.839, -41.9131) ccw
  line L25 (8.5441, -43.2103) -> (8.6422, -43.1908)
  arc A47 (8.6422, -43.1908) -> (11.2302, -43.8996) centre (10.6449, -40.9572) ccw
  arc A48 (11.2302, -43.8996) -> (15.0517, -42.7403) centre (0, 0) ccw
  arc A49 (15.0517, -42.7403) -> (16.8098, -40.7132) centre (13.9037, -39.9686) ccw
  line L26 (16.8098, -40.7132) -> (16.9022, -40.6749)
  arc A50 (16.9022, -40.6749) -> (19.5788, -40.8651) centre (18.4307, -38.0935) ccw
  arc A51 (19.5788, -40.8651) -> (23.1007, -38.9826) centre (0, 0) ccw
  arc A52 (23.1007, -38.9826) -> (24.4296, -36.6515) centre (21.434, -36.4882) ccw
  line L27 (24.4296, -36.6515) -> (24.5127, -36.5959)
  arc A53 (24.5127, -36.5959) -> (27.1749, -36.2603) centre (25.5082, -33.7659) ccw
  arc A54 (27.1749, -36.2603) -> (30.262, -33.7268) centre (0, 0) ccw
  arc A55 (30.262, -33.7268) -> (31.1105, -31.1812) centre (28.1407, -31.6055) ccw
  line L28 (31.1105, -31.1812) -> (31.1812, -31.1105)
  arc A56 (31.1812, -31.1105) -> (33.7268, -30.262) centre (31.6055, -28.1407) ccw
  arc A57 (33.7268, -30.262) -> (36.2603, -27.1749) centre (0, 0) ccw
  arc A58 (36.2603, -27.1749) -> (36.5959, -24.5127) centre (33.7659, -25.5082) ccw
  line L29 (36.5959, -24.5127) -> (36.6515, -24.4296)
  arc A59 (36.6515, -24.4296) -> (38.9826, -23.1007) centre (36.4882, -21.434) ccw
  arc A60 (38.9826, -23.1007) -> (40.8651, -19.5788) centre (0, 0) ccw
  arc A61 (40.8651, -19.5788) -> (40.6749, -16.9022) centre (38.0935, -18.4307) ccw
  line L30 (40.6749, -16.9022) -> (40.7132, -16.8098)
  arc A62 (40.7132, -16.8098) -> (42.7403, -15.0517) centre (39.9686, -13.9037) ccw
  arc A63 (42.7403, -15.0517) -> (43.8996, -11.2302) centre (0, 0) ccw
  arc A64 (43.8996, -11.2302) -> (43.1908, -8.6422) centre (40.9572, -10.6449) ccw
  line L31 (43.1908, -8.6422) -> (43.2103, -8.5441)
  arc A65 (43.2103, -8.5441) -> (44.8555, -6.4243) centre (41.9131, -5.839) ccw
  arc A66 (44.8555, -6.4243) -> (45.2469, -2.45) centre (0, 0) ccw
  arc A67 (45.2469, -2.45) -> (44.0469, -0.05) centre (42.2469, -2.45) ccw
  line L32 (44.0469, -0.05) -> (44.0469, 0.05)
  arc A68 (44.0469, 0.05) -> (45.2469, 2.45) centre (42.2469, 2.45) ccw
  arc A69 (45.2469, 2.45) -> (44.8555, 6.4243) centre (0, 0) ccw
  arc A70 (44.8555, 6.4243) -> (43.2103, 8.5441) centre (41.9131, 5.839) ccw
  line L33 (43.2103, 8.5441) -> (43.1908, 8.6422)
  arc A71 (43.1908, 8.6422) -> (43.8996, 11.2302) centre (40.9572, 10.6449) ccw
  arc A72 (43.8996, 11.2302) -> (42.7403, 15.0517) centre (0, 0) ccw
  arc A73 (42.7403, 15.0517) -> (40.7132, 16.8098) centre (39.9686, 13.9037) ccw
  line L34 (40.7132, 16.8098) -> (40.6749, 16.9022)
  arc A74 (40.6749, 16.9022) -> (40.8651, 19.5788) centre (38.0935, 18.4307) ccw
  arc A75 (40.8651, 19.5788) -> (38.9826, 23.1007) centre (0, 0) ccw
  arc A76 (38.9826, 23.1007) -> (36.6515, 24.4296) centre (36.4882, 21.434) ccw
  line L35 (36.6515, 24.4296) -> (36.5959, 24.5127)
  arc A77 (36.5959, 24.5127) -> (36.2603, 27.1749) centre (33.7659, 25.5082) ccw
  arc A78 (36.2603, 27.1749) -> (33.7268, 30.262) centre (0, 0) ccw
  arc A79 (33.7268, 30.262) -> (31.1812, 31.1105) centre (31.6055, 28.1407) ccw
  line L36 (31.1812, 31.1105) -> (31.1105, 31.1812)
  arc A80 (31.1105, 31.1812) -> (30.262, 33.7268) centre (28.1407, 31.6055) ccw
  arc A81 (30.262, 33.7268) -> (27.1749, 36.2603) centre (0, 0) ccw
  arc A82 (27.1749, 36.2603) -> (24.5127, 36.5959) centre (25.5082, 33.7659) ccw
  line L37 (24.5127, 36.5959) -> (24.4296, 36.6515)
  arc A83 (24.4296, 36.6515) -> (23.1007, 38.9826) centre (21.434, 36.4882) ccw
  arc A84 (23.1007, 38.9826) -> (19.5788, 40.8651) centre (0, 0) ccw
  arc A85 (19.5788, 40.8651) -> (16.9022, 40.6749) centre (18.4307, 38.0935) ccw
  line L38 (16.9022, 40.6749) -> (16.8098, 40.7132)
  arc A86 (16.8098, 40.7132) -> (15.0517, 42.7403) centre (13.9037, 39.9686) ccw
  arc A87 (15.0517, 42.7403) -> (11.2302, 43.8996) centre (0, 0) ccw
  arc A88 (11.2302, 43.8996) -> (8.6422, 43.1908) centre (10.6449, 40.9572) ccw
  line L39 (8.6422, 43.1908) -> (8.5441, 43.2103)
  arc A89 (8.5441, 43.2103) -> (6.4243, 44.8555) centre (5.839, 41.9131) ccw
  arc A90 (6.4243, 44.8555) -> (2.45, 45.2469) centre (0, 0) ccw
  arc A91 (2.45, 45.2469) -> (0.05, 44.0469) centre (2.45, 42.2469) ccw
  line L40 (0.05, 44.0469) -> (-0.05, 44.0469)
  arc A92 (-0.05, 44.0469) -> (-2.45, 45.2469) centre (-2.45, 42.2469) ccw
  arc A93 (-2.45, 45.2469) -> (-6.4243, 44.8555) centre (0, 0) ccw
  arc A94 (-6.4243, 44.8555) -> (-8.5441, 43.2103) centre (-5.839, 41.9131) ccw
  line L41 (-8.5441, 43.2103) -> (-8.6422, 43.1908)
  arc A95 (-8.6422, 43.1908) -> (-11.2302, 43.8996) centre (-10.6449, 40.9572) ccw
  arc A96 (-11.2302, 43.8996) -> (-15.0517, 42.7403) centre (0, 0) ccw
  arc A97 (-15.0517, 42.7403) -> (-16.8098, 40.7132) centre (-13.9037, 39.9686) ccw
  line L42 (-16.8098, 40.7132) -> (-16.9022, 40.6749)
  arc A98 (-16.9022, 40.6749) -> (-19.5788, 40.8651) centre (-18.4307, 38.0935) ccw
  arc A99 (-19.5788, 40.8651) -> (-23.1007, 38.9826) centre (0, 0) ccw
  arc A100 (-23.1007, 38.9826) -> (-24.4296, 36.6515) centre (-21.434, 36.4882) ccw
  line L43 (-24.4296, 36.6515) -> (-24.5127, 36.5959)
  arc A101 (-24.5127, 36.5959) -> (-27.1749, 36.2603) centre (-25.5082, 33.7659) ccw
  arc A102 (-27.1749, 36.2603) -> (-30.262, 33.7268) centre (0, 0) ccw
  arc A103 (-30.262, 33.7268) -> (-31.1105, 31.1812) centre (-28.1407, 31.6055) ccw
  line L44 (-31.1105, 31.1812) -> (-31.1812, 31.1105)
  arc A104 (-31.1812, 31.1105) -> (-33.7268, 30.262) centre (-31.6055, 28.1407) ccw
  arc A105 (-33.7268, 30.262) -> (-36.2603, 27.1749) centre (0, 0) ccw
  arc A106 (-36.2603, 27.1749) -> (-36.5959, 24.5127) centre (-33.7659, 25.5082) ccw
  line L45 (-36.5959, 24.5127) -> (-36.6515, 24.4296)
  arc A107 (-36.6515, 24.4296) -> (-38.9826, 23.1007) centre (-36.4882, 21.434) ccw
  arc A108 (-38.9826, 23.1007) -> (-40.8651, 19.5788) centre (0, 0) ccw
  arc A109 (-40.8651, 19.5788) -> (-40.6749, 16.9022) centre (-38.0935, 18.4307) ccw
  line L46 (-40.6749, 16.9022) -> (-40.7132, 16.8098)
  arc A110 (-40.7132, 16.8098) -> (-42.7403, 15.0517) centre (-39.9686, 13.9037) ccw
  arc A111 (-42.7403, 15.0517) -> (-43.8996, 11.2302) centre (0, 0) ccw
  arc A112 (-43.8996, 11.2302) -> (-43.1908, 8.6422) centre (-40.9572, 10.6449) ccw
  line L47 (-43.1908, 8.6422) -> (-43.2103, 8.5441)
  arc A113 (-43.2103, 8.5441) -> (-44.8555, 6.4243) centre (-41.9131, 5.839) ccw
  arc A114 (-44.8555, 6.4243) -> (-45.2469, 2.45) centre (0, 0) ccw
  arc A115 (-45.2469, 2.45) -> (-44.0469, 0.05) centre (-42.2469, 2.45) ccw
  circle A116 centre (15.1, -31) radius 3.05
  circle A117 centre (15.1, 31) radius 3.05
sketch "Эскиз42" plane through (0, -2, 0) normal (0, -1, 0) x (1, 0, 0)
  line L0 (27, -14.15) -> (-27, -14.15)
  arc A0 (-35, -6.15) -> (-27, -14.15) centre (-27, -6.15) ccw
  line L1 (-35, -6.15) -> (-35, 6.15)
  arc A1 (-27, 14.15) -> (-35, 6.15) centre (-27, 6.15) ccw
  line L2 (-27, 14.15) -> (27, 14.15)
  arc A2 (35, 6.15) -> (27, 14.15) centre (27, 6.15) ccw
  line L3 (35, 6.15) -> (35, -6.15)
  arc A3 (27, -14.15) -> (35, -6.15) centre (27, -6.15) ccw
  circle A4 centre (-15.1, -31) radius 1.65
  circle A5 centre (15.1, -31) radius 1.65
  circle A6 centre (-15.1, 31) radius 1.65
  circle A7 centre (15.1, 31) radius 1.65
  arc A8 (-45.2469, 2.45) -> (-44.0469, 0.05) centre (-42.2469, 2.45) ccw
  line L4 (-44.0469, 0.05) -> (-44.0469, -0.05)
  arc A9 (-44.0469, -0.05) -> (-45.2469, -2.45) centre (-42.2469, -2.45) ccw
  arc A10 (-45.2469, -2.45) -> (-44.8555, -6.4243) centre (0, 0) ccw
  arc A11 (-44.8555, -6.4243) -> (-43.2103, -8.5441) centre (-41.9131, -5.839) ccw
  line L5 (-43.2103, -8.5441) -> (-43.1908, -8.6422)
  arc A12 (-43.1908, -8.6422) -> (-43.8996, -11.2302) centre (-40.9572, -10.6449) ccw
  arc A13 (-43.8996, -11.2302) -> (-42.7403, -15.0517) centre (0, 0) ccw
  arc A14 (-42.7403, -15.0517) -> (-40.7132, -16.8098) centre (-39.9686, -13.9037) ccw
  line L6 (-40.7132, -16.8098) -> (-40.6749, -16.9022)
  arc A15 (-40.6749, -16.9022) -> (-40.8651, -19.5788) centre (-38.0935, -18.4307) ccw
  arc A16 (-40.8651, -19.5788) -> (-38.9826, -23.1007) centre (0, 0) ccw
  arc A17 (-38.9826, -23.1007) -> (-36.6515, -24.4296) centre (-36.4882, -21.434) ccw
  line L7 (-36.6515, -24.4296) -> (-36.5959, -24.5127)
  arc A18 (-36.5959, -24.5127) -> (-36.2603, -27.1749) centre (-33.7659, -25.5082) ccw
  arc A19 (-36.2603, -27.1749) -> (-33.7268, -30.262) centre (0, 0) ccw
  arc A20 (-33.7268, -30.262) -> (-31.1812, -31.1105) centre (-31.6055, -28.1407) ccw
  line L8 (-31.1812, -31.1105) -> (-31.1105, -31.1812)
  arc A21 (-31.1105, -31.1812) -> (-30.262, -33.7268) centre (-28.1407, -31.6055) ccw
  arc A22 (-30.262, -33.7268) -> (-27.1749, -36.2603) centre (0, 0) ccw
  arc A23 (-27.1749, -36.2603) -> (-24.5127, -36.5959) centre (-25.5082, -33.7659) ccw
  line L9 (-24.5127, -36.5959) -> (-24.4296, -36.6515)
  arc A24 (-24.4296, -36.6515) -> (-23.1007, -38.9826) centre (-21.434, -36.4882) ccw
  arc A25 (-23.1007, -38.9826) -> (-19.5788, -40.8651) centre (0, 0) ccw
  arc A26 (-19.5788, -40.8651) -> (-16.9022, -40.6749) centre (-18.4307, -38.0935) ccw
  line L10 (-16.9022, -40.6749) -> (-16.8098, -40.7132)
  arc A27 (-16.8098, -40.7132) -> (-15.0517, -42.7403) centre (-13.9037, -39.9686) ccw
  arc A28 (-15.0517, -42.7403) -> (-11.2302, -43.8996) centre (0, 0) ccw
  arc A29 (-11.2302, -43.8996) -> (-8.6422, -43.1908) centre (-10.6449, -40.9572) ccw
  line L11 (-8.6422, -43.1908) -> (-8.5441, -43.2103)
  arc A30 (-8.5441, -43.2103) -> (-6.4243, -44.8555) centre (-5.839, -41.9131) ccw
  arc A31 (-6.4243, -44.8555) -> (-2.45, -45.2469) centre (0, 0) ccw
  arc A32 (-2.45, -45.2469) -> (-0.05, -44.0469) centre (-2.45, -42.2469) ccw
  line L12 (-0.05, -44.0469) -> (0.05, -44.0469)
  arc A33 (0.05, -44.0469) -> (2.45, -45.2469) centre (2.45, -42.2469) ccw
  arc A34 (2.45, -45.2469) -> (6.4243, -44.8555) centre (0, 0) ccw
  arc A35 (6.4243, -44.8555) -> (8.5441, -43.2103) centre (5.839, -41.9131) ccw
  line L13 (8.5441, -43.2103) -> (8.6422, -43.1908)
  arc A36 (8.6422, -43.1908) -> (11.2302, -43.8996) centre (10.6449, -40.9572) ccw
  arc A37 (11.2302, -43.8996) -> (15.0517, -42.7403) centre (0, 0) ccw
  arc A38 (15.0517, -42.7403) -> (16.8098, -40.7132) centre (13.9037, -39.9686) ccw
  line L14 (16.8098, -40.7132) -> (16.9022, -40.6749)
  arc A39 (16.9022, -40.6749) -> (19.5788, -40.8651) centre (18.4307, -38.0935) ccw
  arc A40 (19.5788, -40.8651) -> (23.1007, -38.9826) centre (0, 0) ccw
  arc A41 (23.1007, -38.9826) -> (24.4296, -36.6515) centre (21.434, -36.4882) ccw
  line L15 (24.4296, -36.6515) -> (24.5127, -36.5959)
  arc A42 (24.5127, -36.5959) -> (27.1749, -36.2603) centre (25.5082, -33.7659) ccw
  arc A43 (27.1749, -36.2603) -> (30.262, -33.7268) centre (0, 0) ccw
  arc A44 (30.262, -33.7268) -> (31.1105, -31.1812) centre (28.1407, -31.6055) ccw
  line L16 (31.1105, -31.1812) -> (31.1812, -31.1105)
  arc A45 (31.1812, -31.1105) -> (33.7268, -30.262) centre (31.6055, -28.1407) ccw
  arc A46 (33.7268, -30.262) -> (36.2603, -27.1749) centre (0, 0) ccw
  arc A47 (36.2603, -27.1749) -> (36.5959, -24.5127) centre (33.7659, -25.5082) ccw
  line L17 (36.5959, -24.5127) -> (36.6515, -24.4296)
  arc A48 (36.6515, -24.4296) -> (38.9826, -23.1007) centre (36.4882, -21.434) ccw
  arc A49 (38.9826, -23.1007) -> (40.8651, -19.5788) centre (0, 0) ccw
  arc A50 (40.8651, -19.5788) -> (40.6749, -16.9022) centre (38.0935, -18.4307) ccw
  line L18 (40.6749, -16.9022) -> (40.7132, -16.8098)
  arc A51 (40.7132, -16.8098) -> (42.7403, -15.0517) centre (39.9686, -13.9037) ccw
  arc A52 (42.7403, -15.0517) -> (43.8996, -11.2302) centre (0, 0) ccw
  arc A53 (43.8996, -11.2302) -> (43.1908, -8.6422) centre (40.9572, -10.6449) ccw
  line L19 (43.1908, -8.6422) -> (43.2103, -8.5441)
  arc A54 (43.2103, -8.5441) -> (44.8555, -6.4243) centre (41.9131, -5.839) ccw
  arc A55 (44.8555, -6.4243) -> (45.2469, -2.45) centre (0, 0) ccw
  arc A56 (45.2469, -2.45) -> (44.0469, -0.05) centre (42.2469, -2.45) ccw
  line L20 (44.0469, -0.05) -> (44.0469, 0.05)
  arc A57 (44.0469, 0.05) -> (45.2469, 2.45) centre (42.2469, 2.45) ccw
  arc A58 (45.2469, 2.45) -> (44.8555, 6.4243) centre (0, 0) ccw
  arc A59 (44.8555, 6.4243) -> (43.2103, 8.5441) centre (41.9131, 5.839) ccw
  line L21 (43.2103, 8.5441) -> (43.1908, 8.6422)
  arc A60 (43.1908, 8.6422) -> (43.8996, 11.2302) centre (40.9572, 10.6449) ccw
  arc A61 (43.8996, 11.2302) -> (42.7403, 15.0517) centre (0, 0) ccw
  arc A62 (42.7403, 15.0517) -> (40.7132, 16.8098) centre (39.9686, 13.9037) ccw
  line L22 (40.7132, 16.8098) -> (40.6749, 16.9022)
  arc A63 (40.6749, 16.9022) -> (40.8651, 19.5788) centre (38.0935, 18.4307) ccw
  arc A64 (40.8651, 19.5788) -> (38.9826, 23.1007) centre (0, 0) ccw
  arc A65 (38.9826, 23.1007) -> (36.6515, 24.4296) centre (36.4882, 21.434) ccw
  line L23 (36.6515, 24.4296) -> (36.5959, 24.5127)
  arc A66 (36.5959, 24.5127) -> (36.2603, 27.1749) centre (33.7659, 25.5082) ccw
  arc A67 (36.2603, 27.1749) -> (33.7268, 30.262) centre (0, 0) ccw
  arc A68 (33.7268, 30.262) -> (31.1812, 31.1105) centre (31.6055, 28.1407) ccw
  line L24 (31.1812, 31.1105) -> (31.1105, 31.1812)
  arc A69 (31.1105, 31.1812) -> (30.262, 33.7268) centre (28.1407, 31.6055) ccw
  arc A70 (30.262, 33.7268) -> (27.1749, 36.2603) centre (0, 0) ccw
  arc A71 (27.1749, 36.2603) -> (24.5127, 36.5959) centre (25.5082, 33.7659) ccw
  line L25 (24.5127, 36.5959) -> (24.4296, 36.6515)
  arc A72 (24.4296, 36.6515) -> (23.1007, 38.9826) centre (21.434, 36.4882) ccw
  arc A73 (23.1007, 38.9826) -> (19.5788, 40.8651) centre (0, 0) ccw
  arc A74 (19.5788, 40.8651) -> (16.9022, 40.6749) centre (18.4307, 38.0935) ccw
  line L26 (16.9022, 40.6749) -> (16.8098, 40.7132)
  arc A75 (16.8098, 40.7132) -> (15.0517, 42.7403) centre (13.9037, 39.9686) ccw
  arc A76 (15.0517, 42.7403) -> (11.2302, 43.8996) centre (0, 0) ccw
  arc A77 (11.2302, 43.8996) -> (8.6422, 43.1908) centre (10.6449, 40.9572) ccw
  line L27 (8.6422, 43.1908) -> (8.5441, 43.2103)
  arc A78 (8.5441, 43.2103) -> (6.4243, 44.8555) centre (5.839, 41.9131) ccw
  arc A79 (6.4243, 44.8555) -> (2.45, 45.2469) centre (0, 0) ccw
  arc A80 (2.45, 45.2469) -> (0.05, 44.0469) centre (2.45, 42.2469) ccw
  line L28 (0.05, 44.0469) -> (-0.05, 44.0469)
  arc A81 (-0.05, 44.0469) -> (-2.45, 45.2469) centre (-2.45, 42.2469) ccw
  arc A82 (-2.45, 45.2469) -> (-6.4243, 44.8555) centre (0, 0) ccw
  arc A83 (-6.4243, 44.8555) -> (-8.5441, 43.2103) centre (-5.839, 41.9131) ccw
  line L29 (-8.5441, 43.2103) -> (-8.6422, 43.1908)
  arc A84 (-8.6422, 43.1908) -> (-11.2302, 43.8996) centre (-10.6449, 40.9572) ccw
  arc A85 (-11.2302, 43.8996) -> (-15.0517, 42.7403) centre (0, 0) ccw
  arc A86 (-15.0517, 42.7403) -> (-16.8098, 40.7132) centre (-13.9037, 39.9686) ccw
  line L30 (-16.8098, 40.7132) -> (-16.9022, 40.6749)
  arc A87 (-16.9022, 40.6749) -> (-19.5788, 40.8651) centre (-18.4307, 38.0935) ccw
  arc A88 (-19.5788, 40.8651) -> (-23.1007, 38.9826) centre (0, 0) ccw
  arc A89 (-23.1007, 38.9826) -> (-24.4296, 36.6515) centre (-21.434, 36.4882) ccw
  line L31 (-24.4296, 36.6515) -> (-24.5127, 36.5959)
  arc A90 (-24.5127, 36.5959) -> (-27.1749, 36.2603) centre (-25.5082, 33.7659) ccw
  arc A91 (-27.1749, 36.2603) -> (-30.262, 33.7268) centre (0, 0) ccw
  arc A92 (-30.262, 33.7268) -> (-31.1105, 31.1812) centre (-28.1407, 31.6055) ccw
  line L32 (-31.1105, 31.1812) -> (-31.1812, 31.1105)
  arc A93 (-31.1812, 31.1105) -> (-33.7268, 30.262) centre (-31.6055, 28.1407) ccw
  arc A94 (-33.7268, 30.262) -> (-36.2603, 27.1749) centre (0, 0) ccw
  arc A95 (-36.2603, 27.1749) -> (-36.5959, 24.5127) centre (-33.7659, 25.5082) ccw
  line L33 (-36.5959, 24.5127) -> (-36.6515, 24.4296)
  arc A96 (-36.6515, 24.4296) -> (-38.9826, 23.1007) centre (-36.4882, 21.434) ccw
  arc A97 (-38.9826, 23.1007) -> (-40.8651, 19.5788) centre (0, 0) ccw
  arc A98 (-40.8651, 19.5788) -> (-40.6749, 16.9022) centre (-38.0935, 18.4307) ccw
  line L34 (-40.6749, 16.9022) -> (-40.7132, 16.8098)
  arc A99 (-40.7132, 16.8098) -> (-42.7403, 15.0517) centre (-39.9686, 13.9037) ccw
  arc A100 (-42.7403, 15.0517) -> (-43.8996, 11.2302) centre (0, 0) ccw
  arc A101 (-43.8996, 11.2302) -> (-43.1908, 8.6422) centre (-40.9572, 10.6449) ccw
  line L35 (-43.1908, 8.6422) -> (-43.2103, 8.5441)
  arc A102 (-43.2103, 8.5441) -> (-44.8555, 6.4243) centre (-41.9131, 5.839) ccw
  arc A103 (-44.8555, 6.4243) -> (-45.2469, 2.45) centre (0, 0) ccw
extrude "Выдавливание1" add sketch "Эскиз3" along normal blind 2
sketch "Эскиз5" plane through (0, 0, 0) normal (0, -1, 0) x (0.7730105, 0, 0.6343933)
  line L0 (5.119, 14.6) -> (5.119, -14.864) construction
  line L1 (5.119, 14.6) -> (22.1616, 14.6) construction
  circle A0 centre (5.119, 14.6) radius 1.5
  circle A1 centre (5.119, -14.864) radius 1.5
  line L2 (5.119, 0) -> (0, 0)
  circle A2 centre (0, 0) radius 36.8469 projected
  line L3 (8.168, 17.66) -> (-36.8469, 17.66)
  line L4 (-36.8469, 17.66) -> (-36.8469, -17.913)
  line L5 (-36.8469, -17.913) -> (8.168, -17.913)
  line L6 (8.168, -17.913) -> (8.168, 17.66)
  line L7 (-43.8397, 4.2676) -> (-43.8299, 4.3671) construction
  line L8 (-43.8397, 4.2676) -> (-43.8397, -4.2676) construction
  dimension "d4" = 29.464
  dimension "d5" = 3
  dimension "d6" = 14.6
  dimension "d7" = 5.119
  dimension "d8" = 3.06
  dimension "d9" = 3.049
  dimension "d10" = 3.049
  constraints: 16 end point, 4 parallel, 3 coincident, 3 perpendicular, 2 centre point, 1 equal radius, 1 point on line, 1 tangent, 1 vertical
  measures "d4" distance from line of L1 L0.end
  measures "d5" diameter of A1
  measures "d6" distance from line of L1 L2.start
  measures "d7" distance from line of L0 L2.end
  measures "d8" distance from line of L3 L0.start
  measures "d9" distance from line of L6 L0.start
  measures "d10" distance from line of L5 L0.end
sketch "Эскиз6" plane through (0, 0, 0) normal (0, -1, 0) x (0.7730105, 0, 0.6343933)
  circle A0 centre (0, 0) radius 36.8469 projected
  arc A1 (-24.3345, 27.6681) -> (24.3345, 27.6681) centre (0, 84.2847) ccw
  arc A2 (24.3345, -27.6681) -> (-24.3345, -27.6681) centre (0, -84.2847) ccw
  arc A3 (28.8177, 22.9616) -> (28.8177, -22.9616) centre (59.4541, 0) ccw
  line L0 (24.3345, 27.6681) -> (-24.3345, 27.6681) construction
  line L1 (-24.3345, -27.6681) -> (24.3345, -27.6681) construction
  line L2 (8.168, 17.66) -> (-36.8469, 17.66) construction
  line L3 (28.8177, 22.9616) -> (28.8177, -22.9616) construction
  line L4 (8.168, -17.913) -> (8.168, 17.66) construction
  line L5 (24.3345, 27.6681) -> (28.8177, 22.9616) construction
  line L6 (28.8177, 22.9616) -> (27.4535, 21.6622) construction
  point P0 (0, 22.66)
  point P1 (21.168, 0)
  dimension "d13" = 5
  dimension "d15" = 6.5
  dimension "d16" = 13
  constraints: 14 point on circle, 10 end point, 3 centre point, 3 parallel, 2 perpendicular, 1 equal radius
  measures "d13" distance from line of L2 point (0, 22.66)
  measures "d15" distance from line of L6 L0.start
  measures "d16" distance from line of L4 point (21.168, 0)